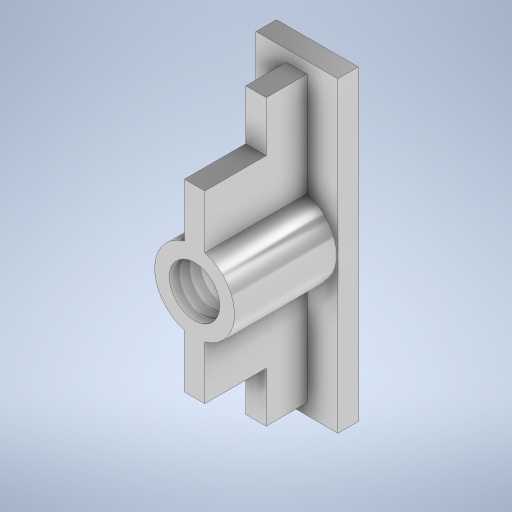
# Autodesk Inventor part: TRAVA
Saved by Autodesk Inventor 2023 (Build 270158000, 158)
## iProperties
Created: 2023-10-18
Part Number: TRAVA
Material: Genérico
Document SubType Name: Modeling
Designer: vinicius.sena
Density: 1 g/cm^3
Appearance: Padrão
Author: vinicius.sena
Autodesk Inventor part; units mm, degrees
ref_plane "YZ Plane" through (0, 0, 0) normal (1, 0, 0) x (0, 1, 0)
ref_plane "XZ Plane" through (0, 0, 0) normal (0, 1, 0) x (-1, 0, 0)
ref_plane "XY Plane" through (0, 0, 0) normal (0, 0, 1) x (1, 0, 0)
sketch "Esboço1" plane through (0, 0, 0) normal (0, 0, 1) x (1, 0, 0)
  line L0 (-2, 7.5) -> (2, 7.5)
  line L1 (2, 7.5) -> (2, -7.5)
  line L2 (2, -7.5) -> (-2, -7.5)
  line L3 (-2, -7.5) -> (-2, 7.5)
  line L4 (-2, 7.5) -> (2, -7.5) construction
  line L5 (2, 7.5) -> (-2, -7.5) construction
  point P0 (0, 0)
  dimension "d0" = 4
  dimension "d1" = 15
  constraints: 12 end point, 2 midpoint, 2 parallel, 1 horizontal, 1 perpendicular
  measures "d0" distance of L1.end L2.end
  measures "d1" distance of L0.end L1.end
extrude "Extrusão1" add sketch "Esboço1" along normal blind 1
sketch "Esboço2" plane through (0, 0, 1) normal (0, 0, 1) x (1, 0, 0)
  line L0 (-1.95, 6.95) -> (1.95, 6.95)
  line L1 (1.95, 6.95) -> (1.95, -6.95)
  line L2 (1.95, -6.95) -> (-1.95, -6.95)
  line L3 (-1.95, -6.95) -> (-1.95, 6.95)
  line L4 (-1.95, 6.95) -> (1.95, -6.95) construction
  line L5 (1.95, 6.95) -> (-1.95, -6.95) construction
  point P0 (0, 0)
  dimension "d4" = 3.9
  dimension "d5" = 13.9
  constraints: 12 end point, 2 midpoint, 2 parallel, 1 horizontal, 1 perpendicular
  measures "d4" distance of L1.end L2.end
  measures "d5" distance of L0.end L1.end
extrude "Extrusão2" add sketch "Esboço2" along normal blind 5
sketch "Esboço3" plane through (0, 0, 6) normal (0, 0, 1) x (1, 0, 0)
  circle A0 centre (0, 0) radius 1.95
  line L0 (1.95, -6.95) -> (-1.95, -6.95) projected
  line L1 (-0.5, 6.95) -> (0.5, 6.95)
  line L2 (0.5, 6.95) -> (0.5, -6.95)
  line L3 (0.5, -6.95) -> (-0.5, -6.95)
  line L4 (-0.5, -6.95) -> (-0.5, 6.95)
  line L5 (-0.5, 6.95) -> (0.5, -6.95) construction
  line L6 (0.5, 6.95) -> (-0.5, -6.95) construction
  line L7 (-1.95, 6.95) -> (1.95, 6.95)
  line L8 (1.95, 6.95) -> (1.95, -6.95)
  line L9 (1.95, -6.95) -> (-1.95, -6.95)
  line L10 (-1.95, -6.95) -> (-1.95, 6.95)
  line L11 (-1.95, 6.95) -> (1.95, -6.95) construction
  line L12 (1.95, 6.95) -> (-1.95, -6.95) construction
  point P0 (-1.95, 0)
  point P1 (-0.5, -1.8848)
  point P2 (-0.5, 1.8848)
  point P3 (1.95, 0)
  point P4 (0.5, 1.8848)
  point P5 (0.5, -1.8848)
  dimension "d8" = 3.9
  dimension "d9" = 1
  constraints: 24 end point, 4 midpoint, 4 parallel, 2 horizontal, 2 perpendicular, 1 centre point, 1 coincident, 1 point on line
  measures "d8" diameter of A0
  measures "d9" distance of L2.end L3.end
extrude "Extrusão3" cut sketch "Esboço3" against normal blind 5 contours L8 L0 L2 A0 | A0 L2 L7 L8 | A0 L10 L7 L4 | L4 L0 L10 A0
sketch "Esboço4" plane through (0, 0, 6) normal (0, 0, 1) x (1, 0, 0)
  line L0 (-0.5, -4.5) -> (0.5, -4.5)
  line L1 (0.5, -4.5) -> (0.5, 4.5)
  line L2 (0.5, 4.5) -> (-0.5, 4.5)
  line L3 (-0.5, 4.5) -> (-0.5, -4.5)
  line L4 (-0.5, -4.5) -> (0.5, 4.5) construction
  line L5 (0.5, -4.5) -> (-0.5, 4.5) construction
  line L6 (0.5, 1.8848) -> (0.5, 6.95) projected
  line L7 (-0.5, -6.95) -> (0.5, -6.95)
  line L8 (0.5, -6.95) -> (0.5, 6.95)
  line L9 (0.5, 6.95) -> (-0.5, 6.95)
  line L10 (-0.5, 6.95) -> (-0.5, -6.95)
  line L11 (-0.5, -6.95) -> (0.5, 6.95) construction
  line L12 (0.5, -6.95) -> (-0.5, 6.95) construction
  point P0 (0, 0)
  dimension "d12" = 1
  dimension "d13" = 9
  constraints: 24 end point, 4 midpoint, 4 parallel, 2 horizontal, 2 perpendicular
  measures "d12" distance of L2.end L1.end
  measures "d13" distance of L1.end L0.end
extrude "Extrusão4" cut sketch "Esboço4" against normal blind 3 contours L0 L8 L7 L10 | L10 L9 L6 L2
sketch "Esboço5" plane through (0, 0, 0) normal (0, 0, -1) x (-1, 0, 0)
  point P0 (0, 0)
  point P1 (0, 0)
  dimension "d23" = 0
  dimension "d24" = 0
  measures "d23" distance of point (0, 0) point (0, 0)
  measures "d24" distance of point (0, 0) point (0, 0)
hole "Furo1" at (0, 0, 0) direction (0, 0, 1) diameter 2.459 end through all thread size "M3x0.5" class "6H" standard "ANSI Metric M Profile"
